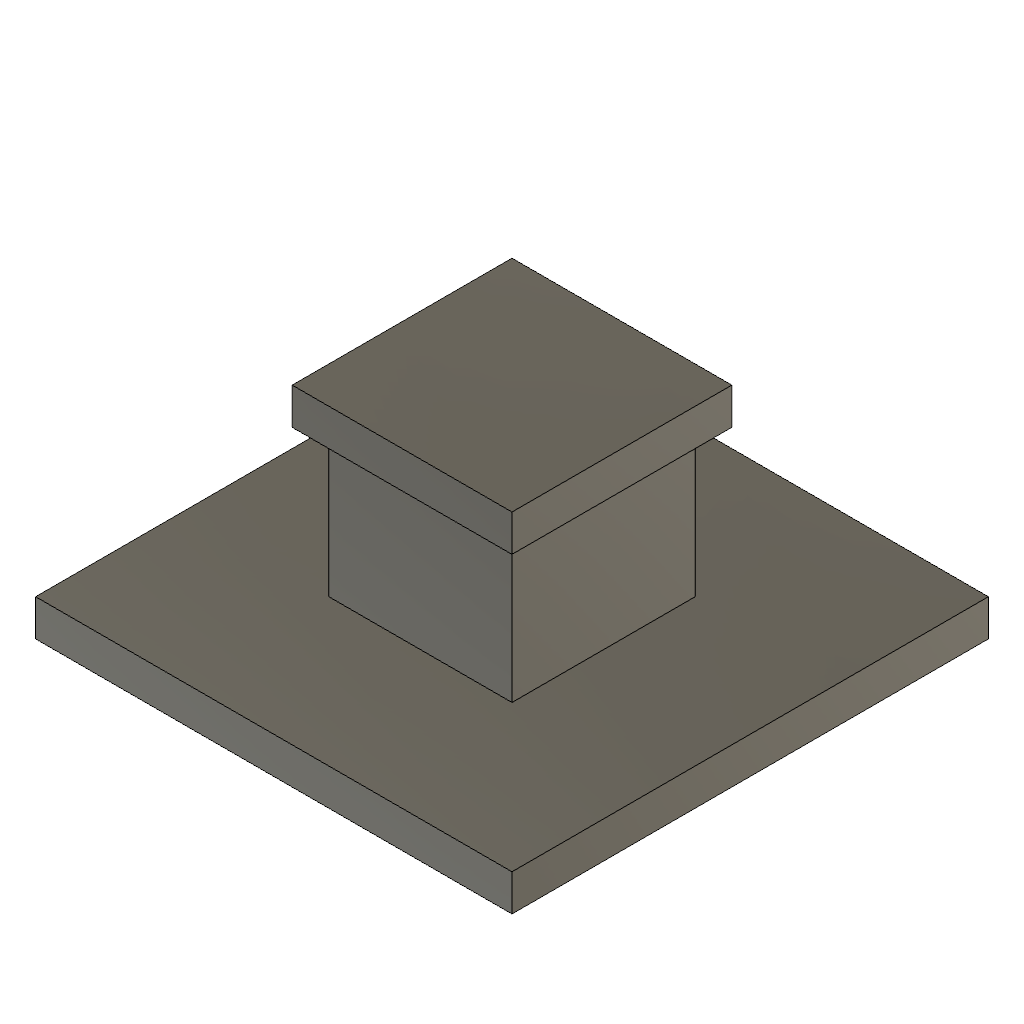
umc-pedestal-g54 (Autodesk Fusion 360 design; units mm, degrees)
part number: 2026-09-12-20-42-12-408
Autodesk Fusion 360 part; units mm, degrees
sketch "Sketch1" plane through (0, 0, 0) normal (0, 0, 1) x (1, 0, 0)
  line L0 (-65, -65) -> (65, -65)
  line L1 (65, -65) -> (65, 65)
  line L2 (65, 65) -> (-65, 65)
  line L3 (-65, 65) -> (-65, -65)
extrude "Extrude1" add sketch "Sketch1" along normal blind 10 from surface at -130 makes body 1
sketch "Sketch2" plane through (0, 0, 0) normal (0, 0, 1) x (1, 0, 0)
  line L0 (-25, -25) -> (25, -25)
  line L1 (25, -25) -> (25, 25)
  line L2 (25, 25) -> (-25, 25)
  line L3 (-25, 25) -> (-25, -25)
extrude "Extrude2" add sketch "Sketch2" along normal blind 40 from surface at -120 separate body makes body 2
sketch "Sketch3" plane through (0, 0, 0) normal (0, 0, 1) x (1, 0, 0)
  line L0 (-30, -30) -> (30, -30)
  line L1 (30, -30) -> (30, 30)
  line L2 (30, 30) -> (-30, 30)
  line L3 (-30, 30) -> (-30, -30)
extrude "Extrude3" add sketch "Sketch3" along normal blind 10 from surface at -80 separate body makes body 3
named bodies: "Mounting base", "Riser", "Top support"
